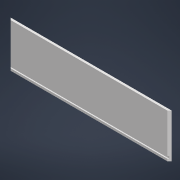
# Autodesk Inventor part: Inert sider
Saved by Autodesk Inventor 2022 (Build 260153000, 153)
## iProperties
Created: 2023-02-16
Part Number: Inert sider
Material: Generic
Document SubType Name: Modeling
Designer: Jakob Saugbjerg
Density: 1 g/cm^3
Appearance: Default
Author: Jakob Saugbjerg
Autodesk Inventor part; units mm, degrees
ref_plane "YZ Plane" through (0, 0, 0) normal (1, 0, 0) x (0, 1, 0)
ref_plane "XZ Plane" through (0, 0, 0) normal (0, 1, 0) x (-1, 0, 0)
ref_plane "XY Plane" through (0, 0, 0) normal (0, 0, 1) x (1, 0, 0)
sketch "Sketch1" plane through (0, 0, 0) normal (0, 0, 1) x (1, 0, 0)
  line L0 (0, 0) -> (220, 0)
  line L1 (220, 0) -> (220, 60)
  line L2 (220, 60) -> (0, 60)
  line L3 (0, 60) -> (0, 0)
  dimension "d0" = 220
  dimension "d1" = 60
  constraints: 8 end point, 2 parallel, 1 horizontal, 1 perpendicular
  measures "d0" distance of L2.end L1.end
  measures "d1" distance of L0.end L1.end
extrude "Extrusion1" add sketch "Sketch1" along normal blind 3
sketch "Sketch2" plane through (0, 0, 3) normal (0, 0, 1) x (1, 0, 0)
  line L0 (0, 60) -> (0, 0) projected
  line L1 (0, 0) -> (0, 3)
  line L2 (0, 0) -> (3, 0) construction
  line L3 (0, 3) -> (220, 3)
  line L4 (220, 3) -> (220, 6)
  line L5 (220, 6) -> (0, 6)
  line L6 (0, 6) -> (0, 3)
  dimension "d4" = 3
  dimension "d5" = 90
  dimension "d6" = 220
  dimension "d7" = 3
  constraints: 12 end point, 2 horizontal, 2 parallel, 2 perpendicular, 1 collinear
  measures "d4" distance of L0.end L1.end
  measures "d5" angle of L2 L1
  measures "d6" distance of L5.end L4.end
  measures "d7" distance of L4.end L3.end
extrude "Extrusion2" cut sketch "Sketch2" against normal blind 1.5
chamfer "Chamfer1" distance 3 angle 45 1 edges at (0, 33, 3)
chamfer "Chamfer2" distance 3 angle 45 1 edges at (220, 33, 3)
body "Solid1"
